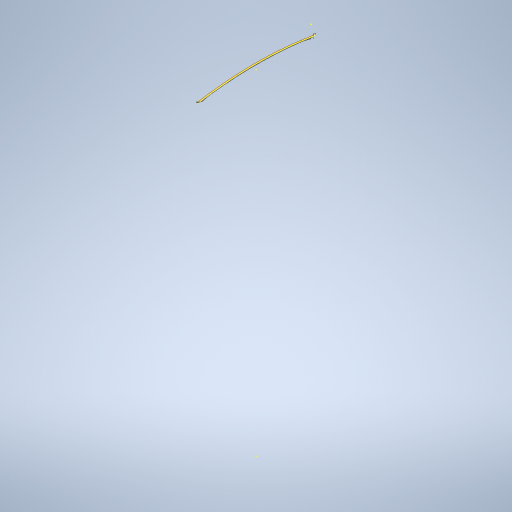
# Autodesk Inventor part: Part1
Saved by Autodesk Inventor 2024.2 (Build 282272000, 272)
## iProperties
Created: 2024-05-18
Part Number: Part1
Material: Wood (Birch)
Document SubType Name: Modeling
Designer: LOSTER_1
Density: 0.55 g/cm^3
Appearance: Birch - Natural Polished
Author: LOSTER_1
Autodesk Inventor part; units mm, degrees
ref_plane "YZ Plane" through (0, 0, 0) normal (1, 0, 0) x (0, 1, 0)
ref_plane "XZ Plane" through (0, 0, 0) normal (0, 1, 0) x (-1, 0, 0)
ref_plane "XY Plane" through (0, 0, 0) normal (0, 0, 1) x (1, 0, 0)
sketch "Sketch1" plane through (0, 0, 0) normal (1, 0, 0) x (0, 1, 0)
  arc A0 (0, -20000) -> (0, 20000) centre (-198997.4874, 0) ccw
  arc A1 (310.8763, 20809.8284) -> (0, 20000) centre (2453.9848, 19522.55) ccw
  arc A2 (310.8763, 20809.8284) -> (329.1509, 20941.157) centre (-568.9757, 20999.1973) ccw
  arc A3 (392.3115, 20998.0517) -> (329.1509, 20941.157) centre (435.8393, 20886.2245) ccw
  line L0 (392.3115, 20998.0517) -> (392.3115, 20788.0517)
  line L1 (392.3115, 20998.0517) -> (602.3115, 20998.0517) construction
  arc A4 (392.3115, 20788.0517) -> (190.7878, 20060) centre (4129.3676, 19361.7237) ccw
  arc A5 (0, -20000) -> (310.8763, -20809.8284) centre (2453.9848, -19522.55) ccw
  arc A6 (329.1509, -20941.157) -> (310.8763, -20809.8284) centre (-568.9757, -20999.1973) ccw
  arc A7 (329.1509, -20941.157) -> (392.3115, -20998.0517) centre (435.8393, -20886.2245) ccw
  line L2 (392.3115, -20998.0517) -> (392.3115, -20788.0517)
  line L3 (392.3115, -20998.0517) -> (602.3115, -20998.0517) construction
  arc A8 (190.7878, -20060) -> (392.3115, -20788.0517) centre (4129.3676, -19361.7237) ccw
  arc A9 (190.7878, -20060) -> (190.7878, 20060) centre (-118120.6503, 0) ccw
  line L4 (190.7878, -20060) -> (0, -20000)
  line L5 (190.7878, 20060) -> (0, 20000)
  point P0 (0, 0)
  point P1 (190, -20060)
  dimension "d0" = 200000
  dimension "d1" = 20000
  dimension "d2" = 20000
  dimension "d3" = 0
  dimension "d4" = 0
  dimension "d5" = 2500
  dimension "d6" = 900
  dimension "d7" = 120
  dimension "d8" = 210
  dimension "d9" = 90
  dimension "d10" = 4000
  dimension "d11" = 200
  dimension "d12" = 60
  dimension "d13" = 120000
  constraints: 20 point on circle, 12 end point, 10 centre point, 1 horizontal, 1 perpendicular, 1 vertical
  measures "d0" radius of A0
  measures "d1" distance of point (0, 0) L5.end
  measures "d2" distance of L4.end point (0, 0)
  measures "d3" horizontal distance of point (0, 0) L5.end
  measures "d4" horizontal distance of point (0, 0) L4.end
  measures "d5" radius of A1
  measures "d6" radius of A2
  measures "d7" radius of A3
  measures "d8" distance of L0.start L0.end
  measures "d9" angle of L0 L1
  measures "d10" radius of A4
  measures "d11" distance of L5.end L5.start
  measures "d12" vertical distance of L5.end L5.start
  measures "d13" radius of A9
extrude "Extrusion1" add sketch "Sketch1" along normal blind 150 and the other way blind 150
sketch "Sketch2" plane through (-150, 392.3115, 20998.0517) normal (0, 1, 0) x (1, 0, 0)
  point P0 (150, 20998.0517)
sketch "Sketch4" plane through (-150, 392.3115, 20998.0517) normal (0, 1, 0) x (1, 0, 0)
  point P0 (150, 20998.0517)
sketch "Sketch5" plane through (-150, 392.3115, 20998.0517) normal (0, 1, 0) x (1, 0, 0)
  point P0 (150, 20998.0517)
sketch "Sketch7" plane through (150, 0, 0) normal (1, 0, 0) x (0, 0, -1)
  arc A0 (-20809.8284, 310.8763) -> (-20000, 0) centre (-19522.55, 2453.9848) ccw projected
  arc A1 (20000, 0) -> (20809.8284, 310.8763) centre (19522.55, 2453.9848) ccw projected
  arc A2 (20000, 0) -> (-20000, 0) centre (0, -198997.4874) ccw projected
  arc A3 (20000, 0) -> (-20000, 0) centre (0, -198997.4874) ccw
  line L0 (20000, 0) -> (-20000, 0)
  point P0 (0, 0)
  constraints: 2 end point, 2 point on circle, 1 centre point, 1 horizontal
extrude "Extrusion2" add sketch "Sketch7" against normal blind 300
sketch "Sketch8" plane through (150, 0, 0) normal (1, 0, 0) x (0, 0, -1)
  line L0 (0, 0) -> (0, 300)
  line L1 (0, 300) -> (17500, 300)
  line L2 (0, 300) -> (-17500, 300)
  line L3 (0, 300) -> (17500, 300) construction
  arc A0 (17500, 300) -> (-17500, 300) centre (0, -128516.7303) ccw
  dimension "d22" = 300
  dimension "d23" = 17500
  dimension "d24" = 90
  dimension "d25" = 17500
  dimension "d26" = 180
  dimension "d27" = 130000
  constraints: 8 end point, 2 horizontal, 2 point on circle, 1 centre point, 1 collinear, 1 perpendicular, 1 vertical
  measures "d22" distance of L0.start L0.end
  measures "d23" distance of L0.end L1.end
  measures "d24" angle of L0 L1
  measures "d25" distance of L0.end L2.end
  measures "d26" angle of L2 L3
  measures "d27" radius of A0
extrude "Extrusion3" cut sketch "Sketch8" against normal blind 300
sketch "Sketch9" plane through (150, 0, 0) normal (1, 0, 0) x (0, 0, -1)
  line L0 (17500, 300) -> (-17500, 300) projected
  arc A0 (17500, 300) -> (-17500, 300) centre (0, -128516.7303) ccw projected
  line L1 (-17500, 300) -> (-19201.3845, 0)
  line L2 (-20000, 0) -> (20000, 0) projected
  line L3 (-17500, 300) -> (-15772.3689, 300) construction
  line L4 (17500, 300) -> (19201.3845, 0)
  line L5 (17500, 300) -> (19227.6311, 300) construction
  line L6 (19201.3845, 0) -> (-19201.3845, 0)
  point P0 (0, 0)
  dimension "d30" = 170
  dimension "d31" = 10
  constraints: 10 end point, 2 equal length, 2 horizontal, 2 point on line, 1 coincident, 1 collinear
  measures "d30" angle of L1 L3
  measures "d31" angle of L4 L5
extrude "Extrusion4" cut sketch "Sketch9" against normal blind 1000 contours L4 L2 L1 L0
sketch "Sketch10" plane through (150, 0, 0) normal (1, 0, 0) x (0, 0, -1)
  point P0 (0, 0)
sketch "Sketch11" plane through (150, 0, 0) normal (1, 0, 0) x (0, 0, -1)
  line L0 (0, 3000) -> (0, -4000)
  line L1 (-19201.3845, 0) -> (-17500, 300) projected
  line L2 (-19201.3845, 0) -> (-19201.3845, -1114.404)
  line L3 (-19201.3845, 0) -> (-18086.9805, 0) construction
  line L4 (-19201.3845, -1114.404) -> (-19201.3845, 1064.8721)
  arc A0 (19937.196, 170.9801) -> (-19937.196, 170.9801) centre (0, -118120.6503) ccw projected
  line L5 (-19201.3845, -239.6685) -> (-16201.3845, -239.6685)
  line L6 (-16201.3845, -239.6685) -> (-16201.3845, -3239.6685)
  line L7 (-16201.3845, -3239.6685) -> (-16201.3845, 2760.3315)
  line L8 (-16201.3845, -239.6685) -> (-8201.3845, -239.6685)
  line L9 (-8201.3845, -239.6685) -> (-8201.3845, -3239.6685)
  line L10 (-8201.3845, -3239.6685) -> (-8201.3845, 2760.3315)
  arc A1 (17500, 300) -> (-17500, 300) centre (0, -128516.7303) ccw projected
  line L11 (-19201.3845, 292.6447) -> (-19201.3845, 0)
  line L12 (-16201.3845, 740.2631) -> (-16201.3845, 469.7618)
  line L13 (-8201.3845, 1558.6666) -> (-8201.3845, 1224.3091)
  line L14 (0, 1839.3497) -> (0, 1483.2697)
  line L15 (-16251.3845, 705.0124) -> (-16151.3845, 705.0124)
  line L16 (-16151.3845, 705.0124) -> (-16151.3845, 505.0124)
  line L17 (-16151.3845, 505.0124) -> (-16251.3845, 505.0124)
  line L18 (-16251.3845, 505.0124) -> (-16251.3845, 705.0124)
  line L19 (-16251.3845, 705.0124) -> (-16151.3845, 505.0124) construction
  line L20 (-16151.3845, 705.0124) -> (-16251.3845, 505.0124) construction
  line L21 (-8251.3845, 1491.4878) -> (-8151.3845, 1491.4878)
  line L22 (-8151.3845, 1491.4878) -> (-8151.3845, 1291.4878)
  line L23 (-8151.3845, 1291.4878) -> (-8251.3845, 1291.4878)
  line L24 (-8251.3845, 1291.4878) -> (-8251.3845, 1491.4878)
  line L25 (-8251.3845, 1491.4878) -> (-8151.3845, 1291.4878) construction
  line L26 (-8151.3845, 1491.4878) -> (-8251.3845, 1291.4878) construction
  line L27 (-50, 1761.3097) -> (50, 1761.3097)
  line L28 (50, 1761.3097) -> (50, 1561.3097)
  line L29 (50, 1561.3097) -> (-50, 1561.3097)
  line L30 (-50, 1561.3097) -> (-50, 1761.3097)
  line L31 (-50, 1761.3097) -> (50, 1561.3097) construction
  line L32 (50, 1761.3097) -> (-50, 1561.3097) construction
  line L33 (19201.3845, 0) -> (17500, 300)
  line L34 (19201.3845, 0) -> (19201.3845, -1114.404)
  line L35 (19201.3845, 0) -> (18086.9805, 0) construction
  line L36 (19201.3845, -1114.404) -> (19201.3845, 1064.8721)
  line L37 (19201.3845, -239.6685) -> (16201.3845, -239.6685)
  line L38 (16201.3845, -239.6685) -> (16201.3845, -3239.6685)
  line L39 (16201.3845, -3239.6685) -> (16201.3845, 2760.3315)
  line L40 (16201.3845, -239.6685) -> (8201.3845, -239.6685)
  line L41 (8201.3845, -239.6685) -> (8201.3845, -3239.6685)
  line L42 (8201.3845, -3239.6685) -> (8201.3845, 2760.3315)
  line L43 (19201.3845, 292.6447) -> (19201.3845, 0)
  line L44 (16201.3845, 740.2631) -> (16201.3845, 469.7618)
  line L45 (8201.3845, 1558.6666) -> (8201.3845, 1224.3091)
  line L46 (16251.3845, 705.0124) -> (16151.3845, 705.0124)
  line L47 (16151.3845, 705.0124) -> (16151.3845, 505.0124)
  line L48 (16151.3845, 505.0124) -> (16251.3845, 505.0124)
  line L49 (16251.3845, 505.0124) -> (16251.3845, 705.0124)
  line L50 (16251.3845, 705.0124) -> (16151.3845, 505.0124) construction
  line L51 (16151.3845, 705.0124) -> (16251.3845, 505.0124) construction
  line L52 (8251.3845, 1491.4878) -> (8151.3845, 1491.4878)
  line L53 (8151.3845, 1491.4878) -> (8151.3845, 1291.4878)
  line L54 (8151.3845, 1291.4878) -> (8251.3845, 1291.4878)
  line L55 (8251.3845, 1291.4878) -> (8251.3845, 1491.4878)
  line L56 (8251.3845, 1491.4878) -> (8151.3845, 1291.4878) construction
  line L57 (8151.3845, 1491.4878) -> (8251.3845, 1291.4878) construction
  point P0 (0, 0)
  point P1 (-16201.3845, 605.0124)
  point P2 (-8201.3845, 1391.4878)
  point P3 (0, 1661.3097)
  point P4 (16201.3845, 605.0124)
  point P5 (8201.3845, 1391.4878)
  dimension "d34" = 7000
  dimension "d35" = 90
  dimension "d36" = 3000
  dimension "d37" = 3000
  dimension "d38" = 6000
  dimension "d39" = 8000
  dimension "d40" = 3000
  dimension "d41" = 6000
  dimension "d42" = 100
  dimension "d43" = 200
  dimension "d44" = 100
  dimension "d45" = 200
  dimension "d46" = 100
  dimension "d47" = 200
  constraints: 114 end point, 29 symmetric about line, 19 point on line, 9 midpoint, 7 perpendicular, 7 point on circle, 6 coincident, 6 parallel, 5 horizontal, 2 collinear, 2 vertical
  measures "d34" distance of L0.start L0.end
  measures "d35" angle of L2 L3
  measures "d36" distance of L5.start L5.end
  measures "d37" distance of L5.end L6.end
  measures "d38" distance of L6.end L7.end
  measures "d39" distance of L5.end L8.end
  measures "d40" distance of L8.end L9.end
  measures "d41" distance of L9.end L10.end
  measures "d42" distance of L16.end L17.end
  measures "d43" distance of L15.end L16.end
  measures "d44" distance of L22.end L23.end
  measures "d45" distance of L21.end L22.end
  measures "d46" distance of L28.end L29.end
  measures "d47" distance of L27.end L28.end
extrude "Extrusion5" cut sketch "Sketch11" against normal blind 300 contours L27 L28 L29 L0 | L0 L29 L30 L27 | L52 L55 L54 L42 | L42 L54 L53 L52 | L21 L22 L23 L10 | L10 L23 L24 L21 | L46 L49 L48 L39 | L39 L48 L47 L46 | L15 L16 L17 L7 | L7 L17 L18 L15
sketch "Sketch12" plane through (150, 0, 0) normal (1, 0, 0) x (0, 0, -1)
  line L0 (-19201.3845, 0) -> (-17500, 300) projected
  line L1 (-19201.3845, 0) -> (-19201.3845, -240.2498)
  line L2 (0, 0) -> (0, 2792.8341)
  arc A0 (17500, 300) -> (-17500, 300) centre (0, -128516.7303) ccw projected
  line L3 (-16251.3845, 505.0124) -> (-16251.3845, 705.0124) projected
  line L4 (-16251.3845, 505.0124) -> (-16251.3845, 442.2919)
  line L5 (19201.3845, 0) -> (17500, 300) projected
  line L6 (19201.3845, 0) -> (19201.3845, -240.2498)
  arc A1 (-16251.3845, 463.4717) -> (-19201.3845, -240.2498) centre (-9612.6521, -33901.1501) ccw
  arc A2 (19201.3845, -240.2498) -> (16251.3845, 463.4717) centre (9612.6521, -33901.1501) ccw
  point P0 (19201.3845, -240.2498)
  point P1 (16251.3845, 463.4717)
  point P2 (-19201.3845, -240.2498)
  dimension "d53" = 35000
  constraints: 8 end point, 6 symmetric about line, 5 point on circle, 3 vertical, 2 centre point, 2 coincident, 1 point on line, 1 other
  measures "d53" radius of A1
extrude "Extrusion7" add sketch "Sketch12" against normal blind 300
sketch "Sketch13" plane through (150, 0, 0) normal (1, 0, 0) x (0, 0, -1)
  arc A0 (20060, 190.7878) -> (-20060, 190.7878) centre (0, -118120.6503) ccw projected
  arc A1 (20060, 190.7878) -> (20788.0517, 392.3115) centre (19361.7237, 4129.3676) ccw projected
  point P0 (0, 0)
  point P1 (20060, 190.7878)
  constraints: 1 coincident
body "Solid1"
